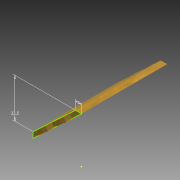
# Autodesk Inventor part: lat_front_mdf2
Saved by Autodesk Inventor 2014 (Build 180170000, 170)
## iProperties
Created: 2015-06-18
Part Number: lat_front_mdf2
Material: Generic
Document SubType Name: Modeling
Designer: Gabriel
Density: 1 g/cm^3
Appearance: Default
Author: Gabriel
Autodesk Inventor part; units mm, degrees
ref_plane "YZ Plane" through (0, 0, 0) normal (1, 0, 0) x (0, 1, 0)
ref_plane "XZ Plane" through (0, 0, 0) normal (0, 1, 0) x (-1, 0, 0)
ref_plane "XY Plane" through (0, 0, 0) normal (0, 0, 1) x (1, 0, 0)
sketch "Sketch1" plane through (0, 0, 0) normal (0, 1, 0) x (-1, 0, 0)
  line L0 (39.6667, 0.3125) -> (0, 37.5)
  line L1 (0, 37.5) -> (5, 37.5)
  line L2 (5, 37.5) -> (39.6667, 5)
  line L3 (39.6667, 5) -> (39.6667, 0.3125)
  point P0 (0, 0)
  dimension "d2" = 5
  dimension "d46" = 32.5
  constraints: 8 end point, 1 parallel
  measures "d2" distance of L0.end L1.end
  measures "d46" distance from line of L2.end L1
extrude "Extrusion1" add sketch "Sketch1" along normal blind 70
sketch "Sketch2" plane through (-39.6667, 0, 0.3125) normal (0.6839411, 0, -0.7295372) x (-0.7295372, 0, -0.6839411)
  line L0 (-54.3406, 0) -> (-29.3406, 0)
  line L1 (-29.3406, 0) -> (-34.3406, 0)
  line L2 (-34.3406, 0) -> (-24.3406, 0)
  line L3 (-28.7246, 0) -> (-30.2246, 0)
  line L4 (-30.2246, 0) -> (-30.2246, 8)
  line L5 (-30.2246, 8) -> (-32.2246, 8)
  line L6 (-32.2246, 8) -> (-32.2246, 13)
  line L7 (-32.2246, 13) -> (-25.2246, 13)
  line L8 (-25.2246, 13) -> (-25.2246, 8)
  line L9 (-25.2246, 8) -> (-27.2246, 8)
  line L10 (-27.2246, 8) -> (-27.2246, 0)
  line L11 (-54.3406, 0) -> (-54.3406, 35)
  line L12 (-54.3406, 35) -> (0.1481, 35)
  line L13 (0.1481, 35) -> (0.1481, 0)
  line L14 (-29.3406, 70) -> (-34.3406, 70)
  line L15 (-34.3406, 70) -> (-24.3406, 70)
  line L16 (-28.7246, 70) -> (-30.2246, 70)
  line L17 (-30.2246, 70) -> (-30.2246, 62)
  line L18 (-30.2246, 62) -> (-32.2246, 62)
  line L19 (-32.2246, 62) -> (-32.2246, 57)
  line L20 (-32.2246, 57) -> (-25.2246, 57)
  line L21 (-25.2246, 57) -> (-25.2246, 62)
  line L22 (-25.2246, 62) -> (-27.2246, 62)
  line L23 (-27.2246, 62) -> (-27.2246, 70)
  dimension "d7" = 25
  dimension "d8" = 5
  dimension "d9" = 10
  dimension "d10" = 1.5
  dimension "d11" = 8
  dimension "d12" = 2
  dimension "d13" = 5
  dimension "d14" = 7
  dimension "d15" = 2
  dimension "d16" = 35
  constraints: 48 end point, 12 symmetric about line, 6 point on line, 5 parallel, 5 perpendicular, 1 horizontal
  measures "d7" distance of L0.start L0.end
  measures "d8" distance of L0.end L1.end
  measures "d9" distance of L1.end L2.end
  measures "d10" distance of L3.start L3.end
  measures "d11" distance of L3.end L4.end
  measures "d12" distance of L4.end L5.end
  measures "d13" distance of L5.end L6.end
  measures "d14" distance of L6.end L7.end
  measures "d15" distance of L8.end L9.end
  measures "d16" distance of L0.start L11.end
extrude "Extrusion2" cut sketch "Sketch2" against normal blind 5 contours L4 L5 L6 L7 L8 L9 L10 L2 L0
extrude "Extrusion3" cut sketch "Sketch2" against normal blind 5 contours L15 L23 L22 L21 L20 L19 L18 L17 L14
sketch "Sketch3" plane through (0, 70, 0) normal (0, 1, 0) x (1, 0, 0)
  line L0 (0, -37.4883) -> (-7.9979, -29.936)
  line L1 (0, -37.4883) -> (-5.022, -37.4883)
  line L2 (-5.022, -37.4883) -> (-45.0001, 0)
  line L3 (0, -37.4883) -> (-7.9979, -29.936)
  line L4 (-7.9979, -29.936) -> (-10.3827, -32.4615)
  line L5 (-10.3827, -32.4615) -> (-16.9476, -26.3054)
  line L6 (-21.8663, -16.9314) -> (-24.2422, -19.4651)
  line L7 (-24.2422, -19.4651) -> (-31.5368, -12.6248)
  line L8 (-31.5368, -12.6248) -> (-29.1608, -10.0911)
  line L9 (-21.8663, -16.9314) -> (-29.1608, -10.0911)
  line L10 (-10.3827, -32.4615) -> (-17.6772, -25.6212)
  line L11 (-7.9979, -29.936) -> (-21.8663, -16.9314)
  line L12 (-17.6772, -25.6212) -> (-15.3013, -23.0875)
  point P0 (0, 0)
  dimension "d25" = 90
  dimension "d28" = 10
  dimension "d32" = 18.4566
  dimension "d33" = 10
  constraints: 26 end point, 6 point on line, 5 perpendicular, 1 collinear, 1 horizontal
  measures "d25" angle of L4 L3
  measures "d28" distance of L6.end L7.end
  measures "d32" distance from line of L2.end L8
  measures "d33" distance of L4.end L10.end
extrude "Extrusion4" add sketch "Sketch3" along normal blind 5 contours L4 L2 L12 L11 | L6 L2 L8 L9
sketch "Sketch4" plane through (0, 0, 0) normal (0, -1, 0) x (1, 0, 0)
  line L0 (0.1144, 37.3726) -> (-7.596, 30.2452)
  line L1 (0.1144, 37.3726) -> (-4.8856, 37.3726)
  line L2 (-4.8856, 37.3726) -> (-44.8855, -0.1225)
  line L3 (-4.8856, 37.3726) -> (-9.8845, 32.6867)
  line L4 (-7.596, 30.2452) -> (-9.8845, 32.6867)
  line L5 (-9.8845, 32.6867) -> (-17.1803, 25.8478)
  line L6 (-17.1803, 25.8478) -> (-14.9244, 23.4411)
  line L7 (-14.9244, 23.4411) -> (-22.2202, 16.6022)
  line L8 (-22.2202, 16.6022) -> (-24.4761, 19.0088)
  line L9 (-24.4761, 19.0088) -> (-31.7719, 12.1699)
  line L10 (-31.7719, 12.1699) -> (-29.6284, 9.8832)
  line L11 (-29.6284, 9.8832) -> (-29.549, 9.7985)
  line L12 (-29.549, 9.7985) -> (-29.5486, 9.7981)
  line L13 (-29.5486, 9.7981) -> (-22.2202, 16.6022)
  line L14 (-14.9244, 23.4411) -> (-7.596, 30.2452)
  point P0 (0, 0)
  constraints: 30 end point, 4 perpendicular, 4 point on line, 2 collinear, 2 parallel, 1 horizontal
extrude "Extrusion5" add sketch "Sketch4" along normal blind 5 contours L14 L6 L2 L4 | L13 L11 L10 L2 L8
body "Solid1"
